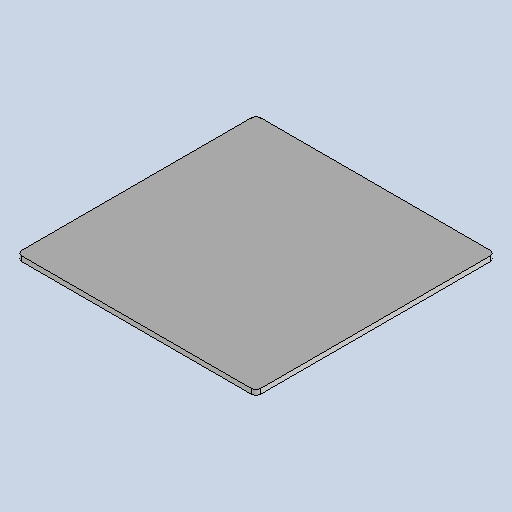
# Autodesk Inventor part: PNS 1665 FDS 1000 CUP 1
Saved by Autodesk Inventor 2025.3 (Build 293356030, 356C)
## iProperties
Created: 2025-06-24
Part Number: PNS 1665 FDS 1000 CUP 1
Material: Stainless Steel
Document SubType Name: Sheet Metal
Designer: admin
Mass: 147.401 g
Surface Area: 191.863 cm^2
Volume: 18.4251 cm^3
Density: 8 g/cm^3
Flat Pattern Width: 9.6 cm
Flat Pattern Length: 9.6 cm
Flat Pattern Area: 92.16 cm^2
Sheet Metal Rule: AISI304 2mm Die16
Sheet Metal Width: 96,000 mm
Sheet Metal Length: 96,000 mm
Sheet Metal Area: 9216,000 mm^2
Appearance: Default
Author: user
Autodesk Inventor part; units mm, degrees
ref_plane "YZ Plane" through (0, 0, 0) normal (1, 0, 0) x (0, 1, 0)
ref_plane "XZ Plane" through (0, 0, 0) normal (0, 1, 0) x (-1, 0, 0)
ref_plane "XY Plane" through (0, 0, 0) normal (0, 0, 1) x (1, 0, 0)
sketch "Sketch1" plane through (0, 0, 0) normal (0, 0, 1) x (1, 0, 0)
  line L0 (-48, -48) -> (48, -48)
  line L1 (48, -48) -> (48, 48)
  line L2 (48, 48) -> (-48, 48)
  line L3 (-48, 48) -> (-48, -48)
  line L4 (-48, -48) -> (48, 48) construction
  line L5 (48, -48) -> (-48, 48) construction
  point P0 (0, 0)
  dimension "d154" = 96
  dimension "d155" = 96
  measures "d154" distance of L1.end L2.end
  measures "d155" distance of L0.end L1.end
extrude "Plate5" add sketch "Sketch1" along normal blind 2
fillet "Corner Round1" radius 2 4 edges at (48, 48, 1) (-48, 48, 1) (-48, -48, 1) (48, -48, 1)
body "Solid3"
